[a]_rubber_foot_block_x4 (Autodesk Fusion 360 design; units mm, degrees)
Autodesk Fusion 360 part; units mm, degrees
sketch "Sketch1" plane through (0, 0, 0) normal (0, 0, 1) x (1, 0, 0)
  line L0 (13, -20) -> (-13, -20)
  line L1 (-13, -20) -> (-13, 20)
  line L2 (-13, 20) -> (13, 20)
  line L3 (13, 20) -> (13, -20)
  line L4 (13, -20) -> (-13, 20) construction
  line L5 (-13, -20) -> (13, 20) construction
  line L6 (0, 20) -> (0, -20)
  circle A0 centre (0, -4) radius 7
  circle A1 centre (0, 10) radius 1.7
  circle A2 centre (0, 10) radius 3
  line L7 (-3.85, 20) -> (-3.85, -20)
  line L8 (3.85, 20) -> (3.85, -20)
  circle A3 centre (0, -4) radius 1.7
  circle A4 centre (0, -4) radius 2.3
  line L9 (-3.85, 15) -> (3.85, 15)
  line L10 (-3.85, 5) -> (3.85, 5)
  line L11 (-3.85, -12) -> (3.85, -12)
  dimension "d1" = 26
  dimension "d2" = 40
  dimension "d3" = 14
  dimension "d4" = 16
  dimension "d5" = 3.4
  dimension "d6" = 6
  dimension "d7" = 7.7
  dimension "d8" = 10
  dimension "d9" = 3.4
  dimension "d10" = 4.6
  dimension "d15" = 5
  dimension "d16" = 5
  dimension "d17" = 8
  constraint horizontal L0
  constraint perpendicular L0 L1
  constraint parallel L0 L2
  constraint parallel L1 L3
  constraint coincident L4 origin
  constraint coincident L5 origin
  constraint midpoint L2 L6.start
  constraint midpoint L0 L6.end
  constraint coincident L6 A0.centre
  constraint coincident L6 A1.centre
  constraint concentric A1 A2
  constraint coincident L2 L7.start
  constraint coincident L0 L7.end
  constraint vertical L7
  constraint symmetric L6 L7.start L8.start
  constraint symmetric L6 L7.end L8.end
  constraint concentric A0 A3
  constraint concentric A3 A4
  constraint coincident L7 L9.start
  constraint coincident L8 L9.end
  constraint horizontal L9
  constraint coincident L7 L10.start
  constraint coincident L8 L10.end
  constraint horizontal L10
  constraint coincident L7 L11.start
  constraint coincident L8 L11.end
  constraint horizontal L11
  measures "d1" distance of L1.end L2.end
  measures "d2" distance of L0.end L1.end
  measures "d3" diameter of A0
  measures "d4" distance of L0 A0.centre
  measures "d5" diameter of A1
  measures "d6" diameter of A2
  measures "d8" distance of L2 A1.centre
  measures "d9" diameter of A3
  measures "d10" diameter of A4
  measures "d15" distance of A1.centre L10
  measures "d16" distance of A1.centre L9
  measures "d17" distance of A0.centre L11
extrude "Extrude1" add sketch "Sketch1" along normal blind 5
extrude "Extrude13" cut sketch "Sketch1" along normal blind 10 contours L6 A3 | L6 A3 | L6 A1 | L6 A1
extrude "Extrude2" add sketch "Sketch1" along normal blind 0.8 from surface at 5 contours L0 L6 L8 L11 | L0 L6 L7 L11 | L2 L6 L8 L9 | L2 L6 L7 L9
fillet "Fillet1" radius 1 8 edges at (-3.85, 20, 5.4) (-3.85, 15, 5.4) (-3.85, -12, 5.4) (-3.85, -20, 5.4) (3.85, -12, 5.4) (3.85, -20, 5.4) (3.85, 15, 5.4) (3.85, 20, 5.4)
chamfer "Chamfer1" distance 0.2 angle 45 16 edges at (3.5571, 15.2929, 5.8) (0, 15, 5.8) (-3.5571, 15.2929, 5.8) (-3.85, 17.5, 5.8) (-3.5571, 19.7071, 5.8) (0, 20, 5.8) (3.5571, 19.7071, 5.8) (3.85, 17.5, 5.8) (3.5571, -19.7071, 5.8) (0, -20, 5.8) (-3.5571, -19.7071, 5.8) (-3.85, -16, 5.8) (-3.5571, -12.2929, 5.8) (0, -12, 5.8) (3.5571, -12.2929, 5.8) (3.85, -16, 5.8)
extrude "Extrude3" cut sketch "Sketch1" along normal blind 3 contours L6 A1 A2 | L6 A1 A2 | L6 A1 | L6 A1
extrude "Extrude5" cut sketch "Sketch1" against normal blind 5 from surface at 5 contours L6 A3 A4 | L6 A3 A4
chamfer "Chamfer3" distance 4 angle 45 4 edges at (13, -20, 2.5) (-13, -20, 2.5) (-13, 20, 2.5) (13, 20, 2.5)
fillet "Fillet2" radius 2 8 edges at (9, -20, 2.5) (-13, 16, 2.5) (13, -16, 2.5) (13, 16, 2.5) (9, 20, 2.5) (-9, 20, 2.5) (-13, -16, 2.5) (-9, -20, 2.5)
chamfer "Chamfer4" distance 0.2 angle 45 20 edges at (-2.1444, -3.1683, 5) (11, 18, 5) (8.9369, 19.8478, 5) (5.5108, 20, 5) (5.5108, -20, 5) (8.9369, -19.8478, 5) (11, -18, 5) (12.8478, -15.9369, 5) (13, 0, 5) (12.8478, 15.9369, 5) (-11, 18, 5) (-12.8478, 15.9369, 5) (-13, 0, 5) (-12.8478, -15.9369, 5) (-11, -18, 5) (-8.9369, -19.8478, 5) (-5.5108, -20, 5) (-5.5108, 20, 5) (-8.9369, 19.8478, 5) (-1.585, 10.6147, 5)
chamfer "Chamfer5" distance 1.5 angle 60 16 edges at (13, 0, 0) (12.8478, -15.9369, 0) (11, -18, 0) (8.9369, -19.8478, 0) (0, -20, 0) (-8.9369, -19.8478, 0) (-11, -18, 0) (-12.8478, -15.9369, 0) (-13, 0, 0) (-12.8478, 15.9369, 0) (-11, 18, 0) (-8.9369, 19.8478, 0) (0, 20, 0) (8.9369, 19.8478, 0) (11, 18, 0) (12.8478, 15.9369, 0) measured on face at (9.4248, -1.2191, 0) measured on face at (12.5321, -16.4571, 1.6) measured on face at (10.5286, -18.4714, 3.2) measured on face at (9.4571, -19.5321, 1.6) measured on face at (9.4248, -1.2191, 0) measured on face at (-8.8556, -19.8794, 1.6) measured on face at (-11.4714, -17.5286, 1.6) measured on face at (-12.6868, -16.2462, 1.6) measured on face at (9.4248, -1.2191, 0) measured on face at (-12.9981, 15.2588, 3.2) measured on face at (-11.4714, 17.5286, 3.2) measured on face at (-8.5189, 19.9696, 3.2) measured on face at (9.4248, -1.2191, 0) measured on face at (9.0168, 19.8126, 1.6) measured on face at (11.4714, 17.5286, 3.2) measured on face at (12.8794, 15.8556, 1.6)
chamfer "Chamfer6" distance 0.4 angle 45 2 edges at (-2.797, 8.9152, 0) (-2.1444, -4.8317, 0) measured on face at (0.0573, -14.4312, 0) measured on face at (0.0573, -14.4312, 0)
sketch "Sketch11" plane through (0, 0, 3) normal (0, 0, -1) x (-1, 0, 0)
  circle A0 centre (0, 10) radius 1.7 construction
  circle A1 centre (0, 10) radius 3
  line L0 (0, 10) -> (1, 10) construction
  line L1 (-2.4712, 8.299) -> (2.4712, 8.299)
  line L2 (-2.4712, 11.701) -> (2.4712, 11.701)
  line L3 (0, 10) -> (0, 8.299) construction
  line L4 (0, 10) -> (0, 11.701) construction
  dimension "d87" = 1.701
  dimension "d88" = 1.701
  constraint coincident A0.centre A1.centre
  constraint parallel L0 L1
  constraint parallel L0 L2
  constraint perpendicular L1 L3
  constraint coincident L1 L3.end
  constraint perpendicular L2 L4
  constraint coincident L2 L4.end
  constraint coincident A1 L1.start
  constraint coincident A1 L1.end
  constraint coincident A1 L2.start
  constraint coincident A1 L2.end
  measures "d87" distance of A0.centre L3.end
  measures "d88" distance of A0.centre L4.end
extrude "Extrude16" cut sketch "Sketch11" against normal blind 0.2 contours A1 L1 L2
sketch "Sketch12" plane through (0, 0, 3.2) normal (0, 0, -1) x (-1, 0, 0)
  circle A0 centre (0, 10) radius 1.7 construction
  line L0 (-2.4712, 8.299) -> (2.4712, 8.299)
  arc A1 (2.4712, 8.299) -> (2.4712, 11.701) centre (0, 10) ccw
  line L1 (2.4712, 11.701) -> (-2.4712, 11.701)
  arc A2 (-2.4712, 11.701) -> (-2.4712, 8.299) centre (0, 10) ccw
  line L2 (0, 10) -> (1, 10) construction
  line L3 (0, 10) -> (0, 11) construction
  line L4 (1.701, 8.299) -> (1.701, 11.701)
  line L5 (-1.701, 8.299) -> (-1.701, 11.701)
  line L6 (0, 10) -> (1.701, 10) construction
  line L7 (0, 10) -> (-1.701, 10) construction
  dimension "d91" = 90
  dimension "d92" = 1.701
  dimension "d93" = 1.701
  constraint coincident A0.centre A1.centre
  constraint parallel L3 L4
  constraint parallel L3 L5
  constraint perpendicular L4 L6
  constraint coincident L4 L6.end
  constraint perpendicular L5 L7
  constraint coincident L5 L7.end
  constraint coincident L0 L4.start
  constraint coincident L1 L4.end
  constraint coincident L0 L5.start
  constraint coincident L1 L5.end
  measures "d91" angle of L2 L3
  measures "d92" distance of A0.centre L6.end
  measures "d93" distance of A0.centre L7.end
extrude "Extrude17" cut sketch "Sketch12" against normal blind 0.2 contours L0 L1 L4 L5
equation "d1 = 30 mm - 4 mm"
equation "d2 = 30 mm + 10 mm"
equation "d7 = 8 mm - 0.3 mm"
equation "d16 = d15"
equation "d17 = ( d3 / 2 ) + 1 mm"
